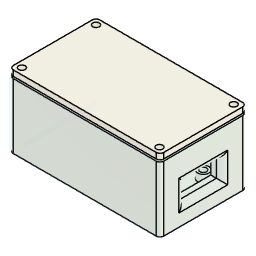
pcb case v3 (Autodesk Fusion 360 design; units mm, degrees)
Autodesk Fusion 360 part; units mm, degrees
note: some values were not read from the file. Chosen so that the rebuilt part matches the saved one: which bodies a step acts on.
sketch "Sketch1" plane through (0, 0, 0) normal (0, 0, 1) x (1, 0, 0)
sketch "Sketch2" plane through (0, 0, 0) normal (0, 0, 1) x (1, 0, 0)
  line L0 (-29, 16) -> (37, 16)
  line L1 (37, 16) -> (37, -16)
  line L2 (37, -16) -> (-29, -16)
  line L3 (-29, -16) -> (-29, 16)
  circle A0 centre (-25, 12) radius 1.75
  circle A1 centre (32, 12) radius 1.75
  circle A2 centre (-24, -12) radius 1.75
  circle A3 centre (33, -12) radius 1.75
  point P0 (-25, 12)
  point P1 (32, 12)
  point P2 (33, -12)
  point P3 (-24, -12)
  point P4 (-25, 12)
  dimension "d6" = 66
  dimension "d7" = 32
  dimension "d8" = 57
  dimension "d9" = 24
  dimension "d10" = 57
  dimension "d11" = 24
  dimension "d12" = 4
  dimension "d13" = 4
  dimension "d14" = 3.5
  dimension "d15" = 3.5
  dimension "d16" = 3.5
  dimension "d17" = 3.5
  constraint horizontal L0
  constraint vertical L1
  constraint horizontal L2
  constraint vertical L3
  constraint coincident P4 P0
  constraint coincident P1 A1.centre
  constraint coincident P3 A2.centre
  constraint coincident P2 A3.centre
  measures "d6" distance of L0.start L0.end
  measures "d7" distance of L0.start L2.end
  measures "d8" distance of P4 P1
  measures "d9" vertical distance of P1 P2
  measures "d10" distance of P2 P3
  measures "d11" vertical distance of P4 P3
  measures "d12" distance of L0 P4
  measures "d13" distance of L2 P2
  measures "d14" diameter of A0
  measures "d15" diameter of A1
  measures "d16" diameter of A2
  measures "d17" diameter of A3
extrude "Extrude1" add sketch "Sketch2" along normal blind 1.6 makes body 1
sketch "Sketch3" plane through (0, 0, 1.6) normal (0, 0, 1) x (-1, 0, 0)
  circle A0 centre (24, 12) radius 1.75
  circle A1 centre (-33, 12) radius 1.75
  circle A2 centre (-32, -12) radius 1.75
  circle A3 centre (25, -12) radius 1.75
  line L0 (29, 16) -> (-37, 16)
  line L1 (-37, 16) -> (-37, -16)
  line L2 (-37, -16) -> (29, -16)
  line L3 (29, -16) -> (29, 16)
  line L4 (32, -19) -> (-40, -19)
  line L5 (-40, -19) -> (-40, 19)
  line L6 (-40, 19) -> (32, 19)
  line L7 (32, 19) -> (32, -19)
  line L8 (30.5, -17.5) -> (-38.5, -17.5)
  line L9 (-38.5, -17.5) -> (-38.5, 17.5)
  line L10 (-38.5, 17.5) -> (30.5, 17.5)
  line L11 (30.5, 17.5) -> (30.5, -17.5)
  circle A4 centre (25, -12) radius 3
  circle A5 centre (24, 12) radius 3
  circle A6 centre (-33, 12) radius 3
  circle A7 centre (-32, -12) radius 3
  point P0 (25, -12)
  point P1 (-32, -12)
  point P2 (-33, 12)
  point P3 (24, 12)
  point P4 (29, -16)
  point P5 (-37, -16)
  point P6 (-37, 16)
  point P7 (29, 16)
  dimension "d20" = 72
  dimension "d21" = 38
  dimension "d22" = 3
  dimension "d23" = 3
  dimension "d24" = 1.5
  dimension "d25" = 1.5
  dimension "d26" = 1.5
  dimension "d27" = 1.5
  dimension "d28" = 6
  constraint horizontal L4
  constraint vertical L5
  constraint horizontal L6
  constraint vertical L7
  constraint coincident P0 A3.centre
  constraint coincident P1 A2.centre
  constraint coincident A1.centre A6.centre
  constraint coincident P3 A0.centre
  constraint coincident P4 L2.end
  constraint coincident P5 L1.end
  constraint coincident L0.end L1.start
  constraint coincident P7 L0.start
  constraint horizontal L8
  constraint vertical L9
  constraint horizontal L10
  constraint vertical L11
  constraint coincident P2 A1.centre
  measures "d20" distance of L4.start L4.end
  measures "d21" distance of L4.start L6.end
  measures "d22" distance of L3 L7
  measures "d23" distance of L2 L4
  measures "d24" distance of L3 L11
  measures "d25" distance of L0 L10
  measures "d26" distance of L1 L9
  measures "d27" distance of L2 L8
  measures "d28" diameter of A7
extrude "Extrude2" add sketch "Sketch3" against normal blind 2 contours L4 L5 L6 L7 | L8 L9 L10 L11 bodies 1
extrude "Extrude3" add 1 faces at (-5.1411, 3.9092, 0) along direction (0, 0, -1) blind 0.5 on bodies 1 bodies 1
extrude "Extrude4" cut 1 faces at (-5.1411, 3.9092, -0.5) along direction (0, 0, 1) blind 0.1 on bodies 1 bodies 1
sketch "Sketch4" plane through (-32, 0, 0) normal (-1, 0, 0) x (0, -1, 0)
  line L0 (19, 1.6) -> (-19, 1.6)
  line L1 (-19, 1.6) -> (-19, -0.4)
  line L2 (-19, -0.4) -> (19, -0.4)
  line L3 (19, -0.4) -> (19, 1.6)
sketch "Sketch5" plane through (0, 0, 1.6) normal (0, 0, 1) x (-1, 0, 0)
  line L0 (32, 19) -> (-40, 19)
  line L1 (-40, 19) -> (-40, -19)
  line L2 (-40, -19) -> (32, -19)
  line L3 (32, -19) -> (32, 19)
  circle A0 centre (24, 12) radius 1.75
  circle A1 centre (-33, 12) radius 1.75
  circle A2 centre (-32, -12) radius 1.75
  circle A3 centre (25, -12) radius 1.75
  line L4 (30, -17) -> (-38, -17)
  line L5 (-38, -17) -> (-38, 17)
  line L6 (-38, 17) -> (30, 17)
  line L7 (30, 17) -> (30, -17)
  circle A4 centre (25, -12) radius 3
  circle A5 centre (-32, -12) radius 3
  circle A6 centre (-33, 12) radius 3
  circle A7 centre (24, 12) radius 3
  line L8 (32, 19) -> (32, -19)
  dimension "d35" = 6
  dimension "d36" = 6
  dimension "d37" = 6
  dimension "d38" = 6
  dimension "d39" = 2
  dimension "d40" = 2
  dimension "d41" = 2
  constraint horizontal L4
  constraint vertical L5
  constraint horizontal L6
  constraint vertical L7
  constraint concentric A3 A4
  constraint concentric A2 A5
  constraint concentric A1 A6
  constraint concentric A0 A7
  measures "d35" diameter of A4
  measures "d36" diameter of A5
  measures "d37" diameter of A6
  measures "d38" diameter of A7
  measures "d39" distance of L2 L4
  measures "d40" distance of L0 L6
  measures "d41" distance of L7 L8
extrude "Extrude5" add sketch "Sketch5" along normal blind 4 contours A4 | A5 | A6 | A7 bodies 1
sketch "Sketch6" plane through (0, 0, 1.6) normal (0, 0, 1) x (-1, 0, 0)
  circle A0 centre (24, 12) radius 3
  circle A1 centre (-32, -12) radius 3
  circle A2 centre (25, -12) radius 3
  circle A3 centre (-33, 12) radius 3
  line L0 (32, 19) -> (-40, 19)
  line L1 (-40, 19) -> (-40, -19)
  line L2 (-40, -19) -> (32, -19)
  line L3 (32, -19) -> (32, 19)
  line L4 (30, -17) -> (-38, -17)
  line L5 (-38, -17) -> (-38, 17)
  line L6 (-38, 17) -> (30, 17)
  line L7 (30, 17) -> (30, -17)
  constraint horizontal L4
  constraint vertical L5
  constraint horizontal L6
  constraint vertical L7
extrude "Extrude6" add sketch "Sketch6" along normal blind 13.5 contours L0 L1 L2 L3 bodies 1
sketch "Sketch7" plane through (-30, 0, 0) normal (1, 0, 0) x (0, 1, 0)
  line L0 (-17, 1.6) -> (17, 1.6)
  line L1 (17, 1.6) -> (17, 15.1)
  line L2 (17, 15.1) -> (-17, 15.1)
  line L3 (-17, 15.1) -> (-17, 1.6)
  line L4 (0, 1.6) -> (0, 5.6)
  line L5 (0, 5.6) -> (0, 7.2)
  line L6 (0, 7.2) -> (5.5, 7.2)
  line L7 (0, 7.2) -> (-5.5, 7.2)
  line L8 (-5.5, 7.2) -> (-5.5, 13.7)
  line L9 (-5.5, 13.7) -> (5.5, 13.7)
  line L10 (5.5, 13.7) -> (5.5, 7.2)
  dimension "d46" = 4
  dimension "d47" = 1.6
  dimension "d48" = 5.5
  dimension "d49" = 5.5
  dimension "d50" = 6.5
  dimension "d51" = 11
  constraint midpoint L0 L4.start
  constraint perpendicular L0 L4
  constraint parallel L4 L5
  constraint perpendicular L5 L6
  constraint perpendicular L5 L7
  constraint perpendicular L7 L8
  constraint perpendicular L8 L9
  measures "d46" distance of L4.start L4.end
  measures "d47" distance of L4.end L5.end
  measures "d48" distance of L5.end L6.end
  measures "d49" distance of L5.end L7.end
  measures "d50" distance of L7.end L8.end
  measures "d51" distance of L8.end L9.end
extrude "Extrude7" cut sketch "Sketch7" against normal blind 2 contours L6 L7 L8 L9 L10 bodies 1
extrude "Extrude8" add 1 faces at (-7.3333, 18.3333, 15.1) along direction (0, 0, 1) blind 17 on bodies 1 bodies 1
sketch "Sketch8" plane through (0, 17, 0) normal (0, -1, 0) x (1, 0, 0)
  line L0 (-30, 1.6) -> (38, 1.6)
  line L1 (38, 1.6) -> (38, 32.1)
  line L2 (38, 32.1) -> (-30, 32.1)
  line L3 (-30, 32.1) -> (-30, 1.6)
  line L4 (0, 1.6) -> (0, 5.6)
  line L5 (0, 5.6) -> (0, 7.2)
  line L6 (0, 18.1) -> (5.45, 18.1)
  line L7 (0, 18.1) -> (-5.45, 18.1)
  line L8 (0, 7.2) -> (5.45, 7.2)
  line L9 (0, 7.2) -> (-5.45, 7.2)
  line L10 (-5.45, 18.1) -> (-5.45, 7.2)
  line L11 (5.45, 18.1) -> (5.45, 7.2)
  dimension "d56" = 4
  dimension "d57" = 1.6
  dimension "d58" = 10.9
  dimension "d59" = 5.45
  dimension "d60" = 5.45
  dimension "d61" = 5.45
  dimension "d62" = 5.45
  constraint coincident L0 L4.start
  constraint perpendicular L0 L4
  constraint parallel L4 L5
  constraint perpendicular L5 L9
  measures "d56" distance of L4.start L4.end
  measures "d57" distance of L4.end L5.end
  measures "d58" distance of L5.end L6.start
  measures "d59" distance of L6.start L6.end
  measures "d60" distance of L6.start L7.end
  measures "d61" distance of L5.end L8.end
  measures "d62" distance of L5.end L9.end
extrude "Extrude9" cut sketch "Sketch8" against normal blind 2 contours L6 L7 L8 L9 L10 L11 bodies 1
extrude "Extrude10" add 1 faces at (16, -19, 21.2667) along direction (0, -1, 0) blind 9 on bodies 1 bodies 1
extrude "Extrude11" add 1 faces at (40, 3.3333, 10.4333) along direction (1, 0, 0) blind 9 on bodies 1 bodies 1
extrude "Extrude12" add 1 faces at (34.4833, 19, 16.6) along direction (0, 1, 0) blind 9 on bodies 1 bodies 1
extrude "Extrude13" add 1 faces at (-32, 1.8333, 25.9667) along direction (-1, 0, 0) blind 9 on bodies 1 bodies 1
sketch "Sketch9" plane through (0, 0, 32.1) normal (0, 0, 1) x (-1, 0, 0)
  line L0 (-38, 17) -> (30, 17)
  line L1 (30, 17) -> (30, -17)
  line L2 (30, -17) -> (-38, -17)
  line L3 (-38, -17) -> (-38, 17)
extrude "Extrude14" add 1 faces at (49, -9.3333, 21.2667) along direction (1, 0, 0) blind 5 on bodies 1 bodies 1
extrude "Extrude15" cut 1 faces at (54, -9.3333, 21.2667) along direction (-1, 0, 0) blind 10 on bodies 1 bodies 1
extrude "Extrude16" cut 1 faces at (-12.6667, -28, 10.4333) along direction (0, 1, 0) blind 5 on bodies 1 bodies 1
extrude "Extrude17" cut 1 faces at (-41, 20.5, 15.1333) along direction (1, 0, 0) blind 5 on bodies 1 bodies 1
extrude "Extrude18" cut 1 faces at (31.15, 28, 16.6) along direction (0, -1, 0) blind 5 on bodies 1 bodies 1
sketch "Sketch10" plane through (0, 0, 32.1) normal (0, 0, 1) x (-1, 0, 0)
sketch "Sketch11" plane through (0, 0, 32.1) normal (0, 0, 1) x (-1, 0, 0)
  circle A0 centre (32.7207, -19.7427) radius 1.75
  circle A1 centre (32.7207, 19.6946) radius 1.75
  circle A2 centre (-40.451, -19.7427) radius 1.75
  circle A3 centre (-40.451, 19.6946) radius 1.75
  point P0 (32.7207, -19.7427)
  point P1 (-40.451, -19.7427)
  point P2 (-40.451, 19.6946)
  point P3 (32.7207, 19.6946)
  dimension "d84" = 3.5
  dimension "d85" = 3.5
  dimension "d86" = 3.5
  dimension "d87" = 3.5
  constraint coincident P0 A0.centre
  constraint coincident P3 A1.centre
  constraint coincident P1 A2.centre
  constraint coincident P2 A3.centre
  measures "d84" diameter of A0
  measures "d85" diameter of A1
  measures "d86" diameter of A2
  measures "d87" diameter of A3
extrude "Extrude19" cut sketch "Sketch11" against normal blind 4 bodies 1
sketch "Sketch12" plane through (0, -23, 0) normal (0, -1, 0) x (1, 0, 0)
  line L0 (-36, 32.1) -> (-36, -0.4)
  line L1 (-36, -0.4) -> (44, -0.4)
  line L2 (44, -0.4) -> (44, 32.1)
  line L3 (44, 32.1) -> (-36, 32.1)
  line L4 (-36, -0.4) -> (44, -0.4)
  line L5 (44, -0.4) -> (44, -2.4)
  line L6 (44, -2.4) -> (-36, -2.4)
  line L7 (-36, -2.4) -> (-36, -0.4)
  dimension "d90" = 2
  constraint horizontal L4
  constraint vertical L5
  constraint horizontal L6
  constraint vertical L7
  constraint coincident L0.end L1.start
  measures "d90" distance of L0.end L6.end
extrude "Extrude20" add sketch "Sketch12" against normal blind 46 contours L1 L4 L5 L6 L7 bodies 1
sketch "Sketch13" plane through (0, -23, 0) normal (0, -1, 0) x (1, 0, 0)
  line L0 (-36, 32.1) -> (-36, -2.4)
  line L1 (-36, -2.4) -> (44, -2.4)
  line L2 (44, -2.4) -> (44, 32.1)
  line L3 (44, 32.1) -> (-36, 32.1)
extrude "Extrude21" add 1 faces at (-7.4232, 19.1723, 32.1) along direction (0, 0, 1) blind 4 on bodies 1 bodies 1
sketch "Sketch14" plane through (0, -23, 0) normal (0, -1, 0) x (1, 0, 0)
  line L0 (-36, 36.1) -> (-36, -2.4)
  line L1 (-36, -2.4) -> (44, -2.4)
  line L2 (44, -2.4) -> (44, 36.1)
  line L3 (44, 36.1) -> (-36, 36.1)
  line L4 (-27.1834, 36.1) -> (-27.1834, 33.1)
  line L5 (-27.1834, 33.1) -> (-36, 33.1)
  line L6 (-27.1834, 33.1) -> (44.0001, 33.1)
  line L7 (-34.7755, 33.1) -> (-34.7755, 32.1)
  line L8 (-34.7755, 32.1) -> (-36, 32.1)
  line L9 (-34.7755, 32.1) -> (44.0121, 32.1)
  dimension "d95" = 3
  dimension "d96" = 1
  constraint coincident L3 L4.start
  constraint perpendicular L3 L4
  constraint coincident L0 L5.end
  constraint perpendicular L0 L5
  constraint perpendicular L2 L6
  constraint coincident L5 L7.start
  constraint perpendicular L5 L7
  constraint coincident L0 L8.end
  constraint perpendicular L0 L8
  constraint perpendicular L2 L9
  measures "d95" distance of L4.start L4.end
  measures "d96" distance of L7.start L7.end
extrude "Extrude22" cut sketch "Sketch14" against normal blind 75 contours L2 L5 L6 L7 L9 bodies 1
sketch "Sketch15" plane through (0, -23, 0) normal (0, -1, 0) x (1, 0, 0)
  line L0 (-27.1834, 33.1) -> (44, 33.1)
  line L1 (44, 33.1) -> (44, 36.1)
  line L2 (44, 36.1) -> (-36, 36.1)
  line L3 (-36, 36.1) -> (-36, -2.4)
  line L4 (-36, -2.4) -> (44, -2.4)
  line L5 (44, -2.4) -> (44, 32.1)
  line L6 (44, 32.1) -> (-34.7755, 32.1)
  line L7 (-34.7755, 32.1) -> (-34.7755, 33.1)
  line L8 (-34.7755, 33.1) -> (-27.1834, 33.1)
  line L9 (-34.7755, 32.1) -> (-36, 32.1)
  line L10 (-34.7755, 33.1) -> (-36, 33.1)
  constraint coincident L6.end L7.start
  constraint coincident L3 L9.end
  constraint perpendicular L3 L9
  constraint coincident L7.end L8.start
  constraint coincident L3 L10.end
  constraint perpendicular L3 L10
extrude "Extrude23" cut sketch "Sketch15" against normal blind 62 contours L3 L7 L9 L10 bodies 1 makes body 2 at (-7.4232, 19.1723, 36.1)
extrude "Extrude24" add 1 faces at (-6.3945, 17, 35.1) along direction (0, -1, 0) blind 34 on bodies 2 bodies 2
fillet "Fillet1" radius 2 1 edges at (-36, -23, 14.85) on bodies 1
fillet "Fillet2" radius 2 5 edges at (-36, 23, 14.85) (44, 23, 14.85) (-36, 23, 34.6) (-36, -23, 34.6) (44, 23, 34.6) on bodies 1 2
fillet "Fillet3" radius 2 1 edges at (44, -23, 34.6) on bodies 2
fillet "Fillet4" radius 2 1 edges at (44, -23, 14.85) on bodies 1
extrude "Extrude25" cut 1 faces at (-1.8167, 19, 7.2) along direction (0, 0, 1) blind 11 on bodies 1 bodies 1
extrude "Extrude26" add 1 faces at (-5.45, 21, 10.8667) along direction (1, 0, 0) blind 10 on bodies 1 bodies 1
extrude "Extrude27" cut 1 faces at (4.55, 21, 10.8667) along direction (1, 0, 0) blind 1 on bodies 1 bodies 1
extrude "Extrude28" add 1 faces at (4.8833, 19, 7.2) along direction (0, 0, 1) blind 11 on bodies 1 bodies 1
sketch "Sketch16" plane through (44, 0, 0) normal (1, 0, 0) x (0, 1, 0)
  line L0 (-21, 32.1) -> (-21, -2.4)
  line L1 (-21, -2.4) -> (21, -2.4)
  line L2 (21, -2.4) -> (21, 32.1)
  line L3 (21, 32.1) -> (-21, 32.1)
move_body "Move1" bodies 2 to x (1, 0, 0) y (0, 1, 0) z (0, 0, 1) at (100, 0, 0)
sketch "Sketch17" plane through (0, 0, 32.1) normal (0, 0, 1) x (-1, 0, 0)
sketch "Sketch18" plane through (44, 0, 0) normal (1, 0, 0) x (0, 1, 0)
sketch "Sketch19" plane through (38, 0, 0) normal (-1, 0, 0) x (0, -1, 0)
  line L0 (17, 32.1) -> (-17, 32.1)
  line L1 (-17, 32.1) -> (-17, 1.6)
  line L2 (-17, 1.6) -> (17, 1.6)
  line L3 (17, 1.6) -> (17, 32.1)
  line L4 (0, 1.6) -> (0, 5.6)
  line L5 (0, 5.6) -> (0, 7.2)
  line L6 (0, 7.2) -> (-10, 7.2)
  line L7 (0, 7.2) -> (10, 7.2)
  line L8 (-10, 7.2) -> (-10, 17.2)
  line L9 (-10, 17.2) -> (10, 17.2)
  line L10 (10, 17.2) -> (10, 7.2)
  dimension "d119" = 4
  dimension "d120" = 1.6
  dimension "d121" = 10
  dimension "d122" = 10
  dimension "d123" = 10
  dimension "d124" = 20
  constraint midpoint L2 L4.start
  constraint perpendicular L2 L4
  constraint parallel L4 L5
  constraint perpendicular L5 L6
  constraint perpendicular L5 L7
  constraint perpendicular L6 L8
  constraint perpendicular L8 L9
  measures "d119" distance of L4.start L4.end
  measures "d120" distance of L4.end L5.end
  measures "d121" distance of L5.end L6.end
  measures "d122" distance of L5.end L7.end
  measures "d123" distance of L6.end L8.end
  measures "d124" distance of L8.end L9.end
extrude "Extrude29" cut sketch "Sketch19" against normal blind 6 contours L6 L7 L8 L9 L10 bodies 1
fillet "Fillet5" radius 3 4 edges at (44, 10, 12.2) (44, 0, 17.2) (44, 0, 7.2) (44, -10, 12.2) on bodies 1
fillet "Fillet6" radius 3 4 edges at (-36, 0, 7.2) (-36, 5.5, 10.45) (-36, 0, 13.7) (-36, -5.5, 10.45) on bodies 1
move_body "Move2" bodies 2 to x (1, 0, 0) y (0, 1, 0) z (0, 0, 1) at (-100, 0, 0)
